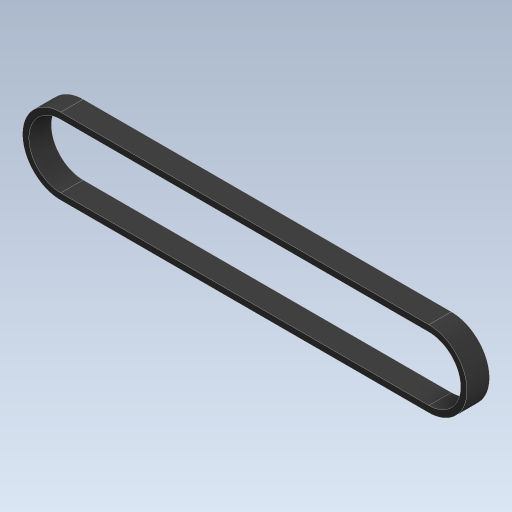
# Autodesk Inventor part: INDX_021_BottomBelt
Saved by Autodesk Inventor 2024 (Build 280153000, 153)
## iProperties
Created: 2024-08-09
Part Number: INDX_021_BottomBelt
Material: Rubber
Document SubType Name: Modeling
Designer: Oscar
Density: 0.93 g/cm^3
Appearance: Rubber - Black
Author: Oscar
Autodesk Inventor part; units mm, degrees
ref_plane "YZ Plane" through (0, 0, 0) normal (1, 0, 0) x (0, 1, 0)
ref_plane "XZ Plane" through (0, 0, 0) normal (0, 1, 0) x (-1, 0, 0)
ref_plane "XY Plane" through (0, 0, 0) normal (0, 0, 1) x (1, 0, 0)
sketch "Sketch1" plane through (0, 0, 0) normal (0, 0, 1) x (1, 0, 0)
  arc A0 (0, 12.7381) -> (0, -12.7381) centre (0, 0) ccw
  arc A1 (147.4978, -12.7381) -> (147.4978, 12.7381) centre (147.4978, 0) ccw
  line L0 (0, 12.7381) -> (147.4978, 12.7381)
  line L1 (147.4978, -12.7381) -> (0, -12.7381)
  line L2 (147.4978, 15.2781) -> (0, 15.2781)
  arc A2 (0, 15.2781) -> (0, -15.2781) centre (0, 0) ccw
  line L3 (0, -15.2781) -> (147.4978, -15.2781)
  arc A3 (147.4978, -15.2781) -> (147.4978, 15.2781) centre (147.4978, 0) ccw
  dimension "d0" = 25.4762
  dimension "d1" = 147.4978
  dimension "d2" = 2.54
  constraints: 8 end point, 8 point on circle, 4 centre point, 4 tangent, 1 coincident, 1 equal radius, 1 horizontal alignment, 3 other
  measures "d0" diameter of A0
  measures "d1" distance of A1.centre A0.centre
  measures "d2" distance between parallel lines of L0 L2
extrude "Extrusion1" add sketch "Sketch1" along normal blind 9
body "Solid1"
